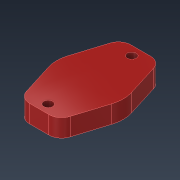
# Autodesk Inventor part: CH_01_0022_bearing_mount
Saved by Autodesk Inventor 2022.3 (Build 263350030, 350C)
## iProperties
Created: 2022-03-04
Part Number: CH_01_0022_bearing_mount
Material: Ogólny
Document SubType Name: Modeling
Designer: zsamot8
Density: 1 g/cm^3
Appearance: Red
Author: zsamot8
Autodesk Inventor part; units mm, degrees
ref_plane "YZ Plane" through (0, 0, 0) normal (1, 0, 0) x (0, 1, 0)
ref_plane "XZ Plane" through (0, 0, 0) normal (0, 1, 0) x (-1, 0, 0)
ref_plane "XY Plane" through (0, 0, 0) normal (0, 0, 1) x (1, 0, 0)
sketch "Szkic1" plane through (0, 0, 0) normal (0, 1, 0) x (-1, 0, 0)
  circle A0 centre (0, 0) radius 11.1
  circle A1 centre (0, 0) radius 13.1
  line L0 (-7.5, 20) -> (7.5, 20)
  line L1 (0, 20) -> (0, 0) construction
  line L2 (7.5, 20) -> (12.5093, 3.8895)
  line L3 (-7.5, 20) -> (-12.5093, 3.8895)
  circle A2 centre (0, 16.5) radius 1.75
  line L4 (0, 0) -> (13.1, 0) construction
  line L5 (-7.5, -20) -> (7.5, -20)
  line L6 (0, -20) -> (0, 0) construction
  line L7 (7.5, -20) -> (12.5093, -3.8895)
  line L8 (-7.5, -20) -> (-12.5093, -3.8895)
  circle A3 centre (0, -16.5) radius 1.75
  arc A4 (12.5093, 3.8895) -> (-12.5093, 3.8895) centre (0, 0) ccw
  arc A5 (-12.5093, -3.8895) -> (12.5093, -3.8895) centre (0, 0) ccw
  dimension "d0" = 22.2
  dimension "d1" = 2
  dimension "d2" = 15
  dimension "d3" = 20
  dimension "d7" = 16.5
  dimension "d8" = 3.5
  constraints: 18 end point, 7 symmetric about line, 6 centre point, 6 point on circle, 5 coincident, 2 point on line, 1 horizontal, 1 midpoint, 1 perpendicular, 1 tangent, 1 vertical, 1 other
  measures "d0" diameter of A0
  measures "d1" radial gap between concentric circles of A1 A0
  measures "d2" distance of L0.start L0.end
  measures "d3" distance of point (0, 0) L1.start
  measures "d7" distance of point (0, 0) A2.centre
  measures "d8" diameter of A2
extrude "Wyciągnięcie proste1" add sketch "Szkic1" along normal blind 7
sketch "Szkic2" plane through (0, 7, 0) normal (0, 1, 0) x (1, 0, 0)
  circle A0 centre (0, 0) radius 13.1
  arc A1 (-12.5093, 3.8895) -> (-12.5093, -3.8895) centre (0, 0) ccw construction
  circle A2 centre (0, 0) radius 10.1
  circle A3 centre (0, 0) radius 11.1 construction
  dimension "d16" = 1
  constraints: 2 centre point, 2 coincident, 1 concentric
  measures "d16" radial gap between concentric circles of A3 A2
extrude "Wyciągnięcie proste2" add sketch "Szkic2" against normal blind 2
fillet "Zaokrąglenie1" radius 5 4 edges at (-7.5, 3.5, 20) (7.5, 3.5, 20) (7.5, 3.5, -20) (-7.5, 3.5, -20)
sketch "Sketch3" plane through (0, 7, 0) normal (0, 1, 0) x (1, 0, 0)
  circle A0 centre (0, 0) radius 10.1 projected
extrude "Extrusion3" add sketch "Sketch3" against normal blind 1
chamfer "Chamfer1" distance 1 angle 45 1 edges at (-10.1, 6, 0)
